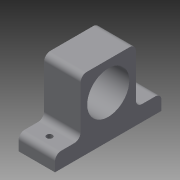
# Autodesk Inventor part: bearing holder
Saved by Autodesk Inventor 2015 (Build 190159000, 159)
## iProperties
Created: 2014-10-25
Part Number: bearing holder
Material: Generic
Document SubType Name: Modeling
Designer: jesse
Density: 1 g/cm^3
Appearance: Default
Author: jesse
Autodesk Inventor part; units mm, degrees
ref_plane "YZ Plane" through (0, 0, 0) normal (1, 0, 0) x (0, 1, 0)
ref_plane "XZ Plane" through (0, 0, 0) normal (0, 1, 0) x (-1, 0, 0)
ref_plane "XY Plane" through (0, 0, 0) normal (0, 0, 1) x (1, 0, 0)
sketch "Sketch1" plane through (0, 0, 0) normal (1, 0, 0) x (0, 1, 0)
  line L0 (0, 4.5482) -> (0, -51.0669)
  line L1 (0, -51.0669) -> (8.138, -51.0669)
  line L2 (8.138, -51.0669) -> (8.138, -37.701)
  line L3 (8.138, -37.701) -> (37.1169, -37.701)
  line L4 (37.1169, -37.701) -> (37.1169, -8.8176)
  line L5 (37.1169, -8.8176) -> (8.138, -8.8176)
  line L6 (8.138, -8.8176) -> (8.138, 4.5482)
  line L7 (8.138, 4.5482) -> (0, 4.5482)
  line L8 (37.1169, -23.2593) -> (0, -23.2593) construction
  circle A0 centre (22.1376, -23.2593) radius 10.9855
  dimension "d0" = 21.971
  constraints: 18 end point, 6 perpendicular, 3 point on line, 2 midpoint, 1 centre point, 1 collinear, 1 vertical
  measures "d0" diameter of A0
extrude "Extrusion1" add sketch "Sketch1" along normal blind 19.05
fillet "Fillet1" radius 3.175 6 edges at (9.525, 37.1169, -8.8176) (9.525, 8.138, -8.8176) (9.525, 37.1169, -37.701) (9.525, 8.138, -37.701) (9.525, 8.138, -51.0669) (9.525, 8.138, 4.5482)
sketch "Sketch2" plane through (0, 8.138, -40.876) normal (0, 1, 0) x (1, 0, 0)
  line L0 (0, 7.0159) -> (19.05, 7.0159) projected
  line L1 (0, 7.0159) -> (0, 0) projected
  line L2 (19.05, 0) -> (0, 0) projected
  line L3 (19.05, 7.0159) -> (19.05, 0) projected
  line L4 (19.05, -42.2493) -> (0, -42.2493) projected
  line L5 (19.05, -35.2334) -> (19.05, -42.2493) projected
  line L6 (0, -35.2334) -> (19.05, -35.2334) projected
  line L7 (0, -35.2334) -> (0, -42.2493) projected
  line L8 (0, 7.0159) -> (19.05, 7.0159) construction
  line L9 (9.525, 7.0159) -> (9.525, 0) construction
  line L10 (0, -35.2334) -> (19.05, -35.2334) construction
  line L11 (9.525, -35.2334) -> (9.525, -42.2493) construction
  circle A0 centre (9.525, 3.5079) radius 1.5356
  circle A1 centre (9.525, -38.7413) radius 1.5356
  point P0 (0, -40.876)
  dimension "d4" = 3.0712
  constraints: 6 midpoint, 4 end point, 2 centre point, 1 equal radius
  measures "d4" diameter of A0
extrude "Extrusion2" cut sketch "Sketch2" against normal through all contours A0 | A1
fillet "Fillet2" radius 1.5875 1 edges at (0, 11.1521, -23.2593)
body "Solid1"
